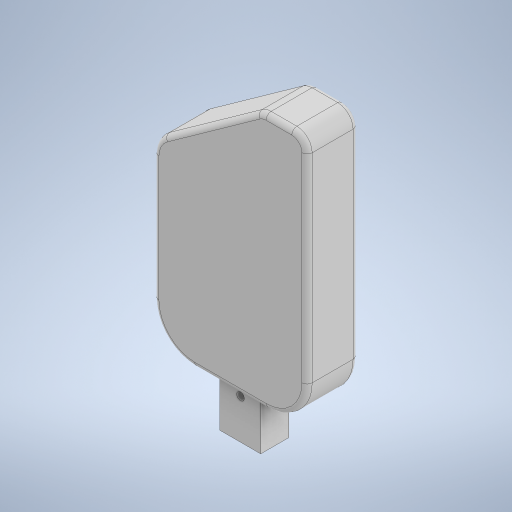
# Autodesk Inventor part: Part1
Saved by Autodesk Inventor 2023.5 (Build 275446020, 446B)
## iProperties
Created: 2025-04-21
Part Number: Part1
Material: Generic
Document SubType Name: Modeling
Designer: Lucky Sah
Density: 1 g/cm^3
Appearance: Default
Author: Lucky Sah
Autodesk Inventor part; units mm, degrees
ref_plane "YZ Plane" through (0, 0, 0) normal (1, 0, 0) x (0, 1, 0)
ref_plane "XZ Plane" through (0, 0, 0) normal (0, 1, 0) x (-1, 0, 0)
ref_plane "XY Plane" through (0, 0, 0) normal (0, 0, 1) x (1, 0, 0)
sketch "Sketch1" plane through (0, 0, 0) normal (0, 0, 1) x (1, 0, 0)
  line L0 (8, 0) -> (22, 0)
  line L1 (30, 8) -> (30, 47)
  line L2 (27, 50) -> (0, 50)
  line L3 (0, 32.4269) -> (0, 8)
  line L4 (0, 50) -> (0, 35)
  line L5 (30, 50) -> (21.9614, 50)
  line L6 (20.2177, 49.4412) -> (2.0938, 36.4956)
  arc A0 (0, 8) -> (8, 0) centre (8, 8) ccw
  arc A1 (22, 0) -> (30, 8) centre (22, 8) ccw
  arc A2 (30, 47) -> (27, 50) centre (27, 47) ccw
  arc A3 (2.0938, 36.4956) -> (0, 32.4269) centre (5, 32.4269) ccw
  arc A4 (21.9614, 50) -> (20.2177, 49.4412) centre (21.9614, 47) ccw
  point P0 (0, 0)
  point P1 (30, 0)
  point P2 (21, 50)
  dimension "d0" = 30
  dimension "d1" = 50
  dimension "d2" = 15
  dimension "d3" = 9
  dimension "d4" = 8
  dimension "d21" = 3
  dimension "d22" = 5
  dimension "d23" = 3
  constraints: 14 end point, 12 point on line, 10 point on circle, 10 tangent, 5 centre point, 2 parallel, 1 equal radius, 1 horizontal, 1 perpendicular
  measures "d0" distance of L2.end L5.start
  measures "d1" distance of L5.start point (30, 0)
  measures "d2" distance of L2.end L4.end
  measures "d3" distance of L5.start point (21, 50)
  measures "d4" radius of A0
  measures "d21" radius of A2
  measures "d22" radius of A3
  measures "d23" radius of A4
extrude "Extrusion1" add sketch "Sketch1" along normal blind 10
fillet "Fillet1" radius 1 14 edges at (2.3431, 2.3431, 10) (15, 0, 10) (27.6569, 2.3431, 10) (30, 27.5, 10) (0, 20.2135, 10) (11.1557, 42.9684, 10) (24.4807, 50, 10) (24.4807, 50, 0) (11.1557, 42.9684, 0) (2.3431, 2.3431, 0) (15, 0, 0) (27.6569, 2.3431, 0) (30, 27.5, 0) (0, 20.2135, 0)
sketch "Sketch2" plane through (8, 0, 9) normal (0, -1, 0) x (1, 0, 0)
  line L0 (4.5, -4.925) -> (9.5, -4.925)
  line L1 (9.5, -4.925) -> (9.5, -2.425)
  line L2 (9.5, -2.425) -> (4.5, -2.425)
  line L3 (4.5, -2.425) -> (4.5, -4.925)
  line L4 (22, -8) -> (22, 0) projected
  line L5 (-8, -8) -> (-8, 0) projected
  line L6 (0, -9) -> (14, -9) projected
  line L7 (14, 1) -> (0, 1) projected
  line L8 (11, -6.425) -> (3, -6.425)
  line L9 (3, -6.425) -> (3, -0.925)
  line L10 (3, -0.925) -> (11, -0.925)
  line L11 (11, -0.925) -> (11, -6.425)
  point P0 (-8, -9)
  dimension "d8" = 5
  dimension "d9" = 2.5
  dimension "d10" = 30
  dimension "d11" = 12.5
  dimension "d12" = 10
  dimension "d13" = 3.425
  dimension "d14" = 1.5
  constraints: 16 end point, 4 parallel, 2 perpendicular, 1 horizontal, 3 other
  measures "d8" distance of L2.end L1.end
  measures "d9" distance of L1.end L0.end
  measures "d10" distance between parallel lines of L4 L5
  measures "d11" distance between parallel lines of L5 L3
  measures "d12" distance between parallel lines of L6 L7
  measures "d13" distance between parallel lines of L7 L2
  measures "d14" distance between parallel lines of L0 L8
extrude "Extrusion2" add sketch "Sketch2" along normal blind 10
sketch "Sketch3" plane through (11, 0, 8.075) normal (0, 0, 1) x (1, 0, 0)
  circle A0 centre (4.0603, -2.2) radius 0.75
  line L0 (8, -10) -> (0, -10) projected
  point P0 (-11, 0)
  dimension "d17" = 1.5
  dimension "d18" = 7.8
  constraints: 1 centre point
  measures "d17" diameter of A0
  measures "d18" distance from line of L0 A0.centre
extrude "Extrusion3" cut sketch "Sketch3" against normal up to surface (5.5 mm away)
body "Solid1"
